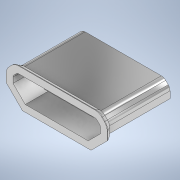
# Autodesk Inventor part: USB Port
Saved by Autodesk Inventor 2020 (Build 240168000, 168)
## iProperties
Created: 2021-03-29
Part Number: USB Port
Material: Generic
Document SubType Name: Modeling
Designer: Luke
Density: 1 g/cm^3
Appearance: Default
Author: Luke
Autodesk Inventor part; units mm, degrees
ref_plane "YZ Plane" through (0, 0, 0) normal (1, 0, 0) x (0, 1, 0)
ref_plane "XZ Plane" through (0, 0, 0) normal (0, 1, 0) x (-1, 0, 0)
sketch "Sketch1" plane through (0, 0, 0) normal (0, 0, 1) x (1, 0, 0)
  line L0 (6.1823, 11.2749) -> (12.3881, 11.2749)
  line L1 (13.0952, 10.5678) -> (13.0952, 10.0149)
  line L2 (11.9552, 8.8749) -> (6.6152, 8.8749)
  line L3 (5.4752, 10.0149) -> (5.4752, 10.5678)
  line L4 (5.4752, 10.0149) -> (6.6152, 8.8749)
  line L5 (11.9552, 8.8749) -> (13.0952, 10.0149)
  line L6 (5.6217, 10.9213) -> (5.8288, 11.1284)
  line L7 (12.7417, 11.1284) -> (12.9488, 10.9213)
  arc A0 (6.1823, 11.2749) -> (5.8288, 11.1284) centre (6.1823, 10.7749) ccw
  arc A1 (5.6217, 10.9213) -> (5.4752, 10.5678) centre (5.9752, 10.5678) ccw
  arc A2 (12.7417, 11.1284) -> (12.3881, 11.2749) centre (12.3881, 10.7749) ccw
  arc A3 (13.0952, 10.5678) -> (12.9488, 10.9213) centre (12.5952, 10.5678) ccw
  line L8 (12.3881, 11.0249) -> (6.1823, 11.0249)
  arc A4 (6.1823, 11.0249) -> (6.0055, 10.9517) centre (6.1823, 10.7749) ccw
  line L9 (6.0055, 10.9517) -> (5.7984, 10.7446)
  arc A5 (5.7984, 10.7446) -> (5.7252, 10.5678) centre (5.9752, 10.5678) ccw
  line L10 (5.7252, 10.5678) -> (5.7252, 10.1184)
  line L11 (5.7252, 10.1184) -> (6.7188, 9.1249)
  line L12 (6.7188, 9.1249) -> (11.8517, 9.1249)
  line L13 (11.8517, 9.1249) -> (12.8452, 10.1184)
  line L14 (12.8452, 10.1184) -> (12.8452, 10.5678)
  arc A6 (12.8452, 10.5678) -> (12.772, 10.7446) centre (12.5952, 10.5678) ccw
  line L15 (12.772, 10.7446) -> (12.5649, 10.9517)
  arc A7 (12.5649, 10.9517) -> (12.3881, 11.0249) centre (12.3881, 10.7749) ccw
  point P0 (0, 0)
  point P1 (13.0952, 8.8749)
  point P2 (5.4752, 8.8749)
  point P3 (5.4752, 11.2749)
  point P4 (13.0952, 11.2749)
  point P5 (5.4752, 10.7749)
  point P6 (5.9752, 11.2749)
  point P7 (12.5952, 11.2749)
  point P8 (13.0952, 10.7749)
  dimension "d0" = 7.62
  dimension "d1" = 2.4
  dimension "d3" = 1.14
  dimension "d4" = 1.14
  dimension "d5" = 1.14
  dimension "d6" = 1.14
  dimension "d7" = 0.5
  dimension "d8" = 0.5
  dimension "d9" = 0.5
  dimension "d10" = 0.5
  dimension "d11" = 0.5
  dimension "d12" = 0.25
  constraints: 32 end point, 16 point on circle, 16 point on line, 8 centre point, 8 tangent, 4 parallel, 3 equal radius, 2 perpendicular, 1 horizontal, 11 other
  measures "d0" distance of point (13.095, 8.875) point (5.475, 8.875)
  measures "d1" distance of point (13.095, 11.275) point (13.095, 8.875)
  measures "d3" distance of L3.start point (5.475, 8.875)
  measures "d4" distance of L2.end point (5.475, 8.875)
  measures "d5" distance of L2.start point (13.095, 8.875)
  measures "d6" distance of L1.end point (13.095, 8.875)
  measures "d7" distance of point (5.475, 10.775) point (5.475, 11.275)
  measures "d8" distance of point (5.975, 11.275) point (5.475, 11.275)
  measures "d9" distance of point (12.595, 11.275) point (13.095, 11.275)
  measures "d10" distance of point (13.095, 10.775) point (13.095, 11.275)
  measures "d11" radius of A0
  measures "d12" distance between parallel lines of L0 L8
extrude "Extrusion1" add sketch "Sketch1" against normal blind 5.42
sketch "Sketch2" plane through (0, 0, -5.42) normal (0, 0, -1) x (-1, 0, 0)
  line L0 (-12.8452, 10.1184) -> (-12.8452, 10.5678) projected
  arc A0 (-12.772, 10.7446) -> (-12.8452, 10.5678) centre (-12.5952, 10.5678) ccw projected
  line L1 (-12.772, 10.7446) -> (-12.5649, 10.9517) projected
  arc A1 (-12.3881, 11.0249) -> (-12.5649, 10.9517) centre (-12.3881, 10.7749) ccw projected
  line L2 (-12.3881, 11.0249) -> (-6.1823, 11.0249) projected
  line L3 (-11.8517, 9.1249) -> (-12.8452, 10.1184) projected
  line L4 (-6.7188, 9.1249) -> (-11.8517, 9.1249) projected
  line L5 (-5.7252, 10.1184) -> (-6.7188, 9.1249) projected
  line L6 (-5.7252, 10.5678) -> (-5.7252, 10.1184) projected
  arc A2 (-5.7252, 10.5678) -> (-5.7984, 10.7446) centre (-5.9752, 10.5678) ccw projected
  arc A3 (-6.0055, 10.9517) -> (-6.1823, 11.0249) centre (-6.1823, 10.7749) ccw projected
  line L7 (-6.0055, 10.9517) -> (-5.7984, 10.7446) projected
extrude "Extrusion2" add sketch "Sketch2" against normal blind 0.2
sketch "Sketch3" plane through (0, 0, -5.22) normal (0, 0, 1) x (1, 0, 0)
  line L0 (7.2852, 10.7249) -> (11.2852, 10.7249)
  line L1 (11.2852, 10.7249) -> (11.2852, 10.0149)
  line L2 (11.2852, 10.0149) -> (7.2852, 10.0149)
  line L3 (7.2852, 10.0149) -> (7.2852, 10.7249)
  line L4 (6.1823, 11.0249) -> (12.3881, 11.0249) projected
  line L5 (9.2852, 11.0249) -> (9.2852, 10.7249)
  point P0 (9.2852, 10.3699)
  point P1 (9.2852, 10.7249)
  dimension "d17" = 4
  dimension "d18" = 0.71
  dimension "d19" = 0.3
  constraints: 10 end point, 2 midpoint, 2 parallel, 1 horizontal, 1 perpendicular, 1 vertical
  measures "d17" distance of L1.end L2.end
  measures "d18" distance of L0.end L1.end
  measures "d19" distance of L5.start L5.end
extrude "Extrusion3" add sketch "Sketch3" along normal blind 4.25
ref_plane "Work Plane1" through (9.2852, 10.0149, 0) normal (-1, 0, 0) x (0, 0, 1)
sketch "Sketch4" plane through (0, 0, 0) normal (0, 0, 1) x (1, 0, 0)
  arc A0 (5.6217, 10.9213) -> (5.4752, 10.5678) centre (5.9752, 10.5678) ccw
  line L0 (5.4752, 10.5678) -> (5.4752, 10.0149)
  line L1 (5.4752, 10.0149) -> (6.6152, 8.8749)
  line L2 (6.6152, 8.8749) -> (11.9552, 8.8749)
  line L3 (11.9552, 8.8749) -> (13.0952, 10.0149)
  line L4 (13.0952, 10.0149) -> (13.0952, 10.5678)
  arc A1 (13.0952, 10.5678) -> (12.9488, 10.9213) centre (12.5952, 10.5678) ccw
  line L5 (12.9488, 10.9213) -> (12.7417, 11.1284)
  arc A2 (12.7417, 11.1284) -> (12.3881, 11.2749) centre (12.3881, 10.7749) ccw
  line L6 (12.3881, 11.2749) -> (6.1823, 11.2749)
  arc A3 (6.1823, 11.2749) -> (5.8288, 11.1284) centre (6.1823, 10.7749) ccw
  line L7 (5.8288, 11.1284) -> (5.6217, 10.9213)
  line L8 (6.1823, 11.5749) -> (12.3881, 11.5749)
  arc A4 (12.9538, 11.3406) -> (12.3881, 11.5749) centre (12.3881, 10.7749) ccw
  line L9 (12.9538, 11.3406) -> (13.1609, 11.1335)
  arc A5 (13.3952, 10.5678) -> (13.1609, 11.1335) centre (12.5952, 10.5678) ccw
  line L10 (13.3952, 10.5678) -> (13.3952, 9.8906)
  line L11 (13.3952, 9.8906) -> (12.0795, 8.5749)
  line L12 (12.0795, 8.5749) -> (6.491, 8.5749)
  line L13 (6.491, 8.5749) -> (5.1752, 9.8906)
  line L14 (5.1752, 9.8906) -> (5.1752, 10.5678)
  arc A6 (5.4095, 11.1335) -> (5.1752, 10.5678) centre (5.9752, 10.5678) ccw
  line L15 (5.4095, 11.1335) -> (5.6166, 11.3406)
  arc A7 (6.1823, 11.5749) -> (5.6166, 11.3406) centre (6.1823, 10.7749) ccw
  dimension "d22" = 0.3
  constraints: 32 end point, 16 point on circle, 12 centre point, 11 other
  measures "d22" distance between parallel lines of L6 L8
extrude "Extrusion4" add sketch "Sketch4" against normal blind 0.4
chamfer "Chamfer1" distance 0.2 angle 60 12 edges at (12.6943, 11.514, -0.4) (13.0573, 11.237, -0.4) (13.3343, 10.8739, -0.4) (13.3952, 10.2292, -0.4) (9.2852, 11.5749, -0.4) (5.8762, 11.514, -0.4) (5.5131, 11.237, -0.4) (5.2361, 10.8739, -0.4) (5.1752, 10.2292, -0.4) (12.7373, 9.2328, -0.4) (5.8331, 9.2328, -0.4) (9.2852, 8.5749, -0.4) measured on face at (10.3195, 11.4749, -0.4)
equation "\"d4\" = d3"
equation "\"d5\" = d3"
equation "\"d6\" = d5"
equation "\"d8\" = d7"
equation "\"d9\" = d7"
equation "\"d10\" = d9"
body "Solid1"
